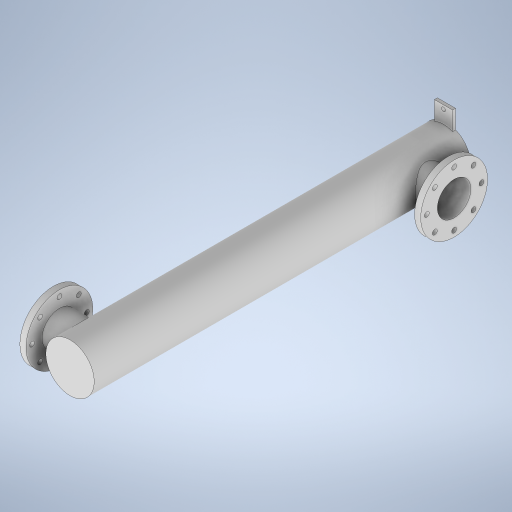
# Autodesk Inventor part: UV-Cleaner ODV-8C
Saved by Autodesk Inventor 2023.2 (Build 272271030, 271C)
## iProperties
Created: 2023-04-12
Part Number: UV-Cleaner ODV-8C
Material: Generic
Document SubType Name: Modeling
Designer: user
Density: 1 g/cm^3
Appearance: Default
Author: user
Autodesk Inventor part; units mm, degrees
ref_plane "YZ Plane" through (0, 0, 0) normal (1, 0, 0) x (0, 1, 0)
ref_plane "XZ Plane" through (0, 0, 0) normal (0, 1, 0) x (-1, 0, 0)
ref_plane "XY Plane" through (0, 0, 0) normal (0, 0, 1) x (1, 0, 0)
sketch "Sketch1" plane through (0, 0, 0) normal (0, 0, 1) x (1, 0, 0)
  line L0 (-30, 135) -> (30, 135)
  line L1 (30, 135) -> (30, 35)
  line L2 (30, 35) -> (-30, 35)
  line L3 (-30, 35) -> (-30, 135)
  line L4 (119.0409, 377.068) -> (884.0572, 377.068) construction
  line L5 (884.0572, 377.068) -> (884.0572, -61.283) construction
  line L6 (884.0572, -61.283) -> (119.0409, -61.283) construction
  line L7 (119.0409, -61.283) -> (119.0409, 377.068) construction
  line L8 (528.2997, 310.003) -> (528.2997, 129.9198)
  line L9 (528.2997, 219.9614) -> (642.893, 286.807)
  circle A0 centre (0, 122) radius 6.5
  point P0 (0, 0)
  point P1 (0, 35)
  point P2 (0, 135)
  dimension "d9" = 60
  dimension "d10" = 100
  dimension "d13" = 135
  dimension "d14" = 13
  dimension "d15" = 13
  constraints: 12 end point, 3 midpoint, 2 parallel, 2 vertical alignment, 1 centre point, 1 horizontal, 1 perpendicular, 1 vertical, 2 other
  measures "d9" distance of L0.start L0.end
  measures "d10" distance of L2.end L0.start
  measures "d13" distance from line of point (0, 0) L0
  measures "d14" diameter of A0
  measures "d15" distance from line of L0 A0.centre
extrude "Extrusion1" add sketch "Sketch1" along normal blind 10
pattern_circular "Circular Pattern1" count 3 over 360 about axis through (0, 0, -10) along (0, 0, 1) of "Extrusion1"
sketch "Sketch2" plane through (0, 0, 0) normal (0, 0, 1) x (1, 0, 0)
  circle A0 centre (0, 0) radius 79.5
  dimension "d21" = 159
  constraints: 1 centre point, 1 coincident
  measures "d21" diameter of A0
extrude "Extrusion2" add sketch "Sketch2" along normal blind 1240
sketch "Sketch3" plane through (0, 0, 0) normal (1, 0, 0) x (0, 1, 0)
  circle A0 centre (0, 125) radius 57
  circle A1 centre (0, 125) radius 55
  point P0 (0, 0)
  dimension "d24" = 114
  dimension "d25" = 125
  dimension "d112" = 2
  constraints: 2 centre point, 1 vertical alignment
  measures "d24" diameter of A0
  measures "d25" distance of point (0, 0) A0.centre
  measures "d112" radial gap between concentric circles of A0 A1
extrude "Extrusion3" add sketch "Sketch3" along normal blind 150
sketch "Sketch4" plane through (0, 0, 0) normal (1, 0, 0) x (0, 1, 0)
  circle A0 centre (0, 1145) radius 57
  line L0 (508.6061, 725.4056) -> (1697.4131, 725.4056) construction
  line L1 (1697.4131, 725.4056) -> (1697.4131, 178.9914) construction
  line L2 (1697.4131, 178.9914) -> (508.6061, 178.9914) construction
  line L3 (508.6061, 178.9914) -> (508.6061, 725.4056) construction
  line L4 (1437.8763, 515.5441) -> (1697.4131, 515.5441)
  line L5 (1697.4131, 515.5441) -> (1697.4131, 335.5441)
  line L6 (1697.4131, 335.5441) -> (1437.8763, 335.5441)
  line L7 (1437.8763, 335.5441) -> (1437.8763, 515.5441)
  line L8 (1526.1756, 486.7469) -> (1616.156, 486.7469)
  line L9 (73.6223, 0) -> (73.6223, 10) projected
  line L10 (73.6223, 0) -> (-10.8304, 0) projected
  line L11 (-10.8304, 10) -> (-10.8304, 0) projected
  line L12 (-62.7919, 10) -> (-10.8304, 10) projected
  line L13 (-62.7919, 0) -> (-62.7919, 10) projected
  line L14 (-62.7919, 0) -> (-62.7919, 0) projected
  line L15 (-62.7919, 10) -> (-62.7919, 0) projected
  line L16 (-10.8304, 10) -> (-62.7919, 10) projected
  line L17 (-10.8304, 0) -> (-10.8304, 10) projected
  line L18 (-10.8304, 0) -> (73.6223, 0) projected
  line L19 (73.6223, 10) -> (73.6223, 0) projected
  line L20 (73.6223, 10) -> (73.6223, 10) projected
  line L21 (79.5, 1240) -> (-79.5, 1240) projected
  circle A1 centre (0, 1145) radius 55
  point P0 (0, 0)
  point P1 (57, 125)
  dimension "d28" = 114
  dimension "d29" = 1145
  dimension "d71" = 180
  dimension "d90" = 89.9804
  dimension "d93" = 95
  dimension "d103" = 2
  constraints: 10 end point, 2 centre point, 2 horizontal, 2 parallel, 1 perpendicular, 1 point on line, 1 vertical alignment, 3 other
  measures "d28" diameter of A0
  measures "d29" distance of point (0, 0) A0.centre
  measures "d71" distance of L6.end L4.start
  measures "d90" distance of L8.start L8.end
  measures "d93" distance from line of A0.centre L21
  measures "d103" radial gap between concentric circles of A0 A1
extrude "Extrusion4" add sketch "Sketch4" against normal blind 150 contours A0
sketch "Sketch5" plane through (-150, 0, 1145) normal (-1, 0, 0) x (0, 0, 1)
  circle A0 centre (0, 0) radius 57 projected
  circle A1 centre (0, 0) radius 110
  circle A2 centre (0, 0) radius 90 construction
  circle A3 centre (90, 0) radius 8
  circle A4 centre (63.6396, 63.6396) radius 8
  circle A5 centre (0, 90) radius 8
  circle A6 centre (-63.6396, 63.6396) radius 8
  circle A7 centre (-90, 0) radius 8
  circle A8 centre (-63.6396, -63.6396) radius 8
  circle A9 centre (0, -90) radius 8
  circle A10 centre (63.6396, -63.6396) radius 8
  point P0 (-1145, 0)
  dimension "d95" = 180
  dimension "d94" = 220
  dimension "d96" = 16
  dimension "d99" = 360
  constraints: 9 centre point, 2 coincident, 2 horizontal alignment, 19 other
  measures "d94" diameter of A1
  measures "d96" diameter of A3
extrude "Extrusion5" add sketch "Sketch5" against normal blind 20
sketch "Sketch6" plane through (150, 0, 125) normal (1, 0, 0) x (0, 0, -1)
  circle A0 centre (0, 0) radius 110
  circle A1 centre (0, 0) radius 90 construction
  circle A2 centre (-90, 0) radius 8
  circle A3 centre (-63.6396, -63.6396) radius 8
  circle A4 centre (0, -90) radius 8
  circle A5 centre (63.6396, -63.6396) radius 8
  circle A6 centre (90, 0) radius 8
  circle A7 centre (63.6396, 63.6396) radius 8
  circle A8 centre (0, 90) radius 8
  circle A9 centre (-63.6396, 63.6396) radius 8
  circle A10 centre (0, 0) radius 57 projected
  point P0 (125, 0)
  dimension "d107" = 180
  dimension "d106" = 220
  dimension "d108" = 16
  dimension "d109" = 360
  constraints: 9 centre point, 3 coincident, 2 horizontal alignment, 19 other
  measures "d106" diameter of A0
  measures "d108" diameter of A2
extrude "Extrusion6" add sketch "Sketch6" against normal blind 20
equation "\"d21\" = main_diameter"
equation "\"d22\" = main_height"
equation "\"d24\" = connect_pipe"
equation "\"d28\" = connect_pipe"
equation "\"main_height\" = 1240"
equation "\"connect_pipe\" = 114"
equation "\"main_diameter\" = 159"
body "Solid1"
